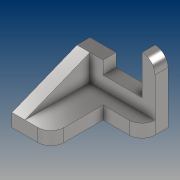
# Autodesk Inventor part: 5
Saved by Autodesk Inventor 2020.2 (Build 242310000, 310)
## iProperties
Created: 2020-09-17
Part Number: 5
Material: 鋼、碳鋼
Document SubType Name: Modeling
Designer: user
Density: 7.85 g/cm^3
Appearance: 半拋光
Mass: 308.946 g
Surface Area: 109.81 cm^2
Volume: 39.3562 cm^3
Author: user
Autodesk Inventor part; units mm, degrees
ref_plane "YZ Plane" through (0, 0, 0) normal (1, 0, 0) x (0, 1, 0)
ref_plane "XZ Plane" through (0, 0, 0) normal (0, 1, 0) x (-1, 0, 0)
ref_plane "XY Plane" through (0, 0, 0) normal (0, 0, 1) x (1, 0, 0)
sketch "草圖1" plane through (0, 0, 0) normal (0, 1, 0) x (-1, 0, 0)
  line L0 (0, 0) -> (0, 60)
  line L1 (-60, 10) -> (-60, 0)
  line L2 (-60, 0) -> (0, 0)
  line L3 (0, 60) -> (-20, 60)
  arc A0 (-20, 60) -> (-30, 50) centre (-20, 50) ccw
  line L4 (-30, 50) -> (-30, 20)
  line L5 (-30, 20) -> (-50, 20)
  arc A1 (-50, 20) -> (-60, 10) centre (-50, 10) ccw
  dimension "d0" = 60
  dimension "d1" = 10
  dimension "d2" = 20
  dimension "d3" = 60
  dimension "d4" = 30
  dimension "d5" = 20
  constraints: 12 end point, 4 point on circle, 4 tangent, 2 centre point, 2 horizontal, 2 perpendicular, 2 vertical
  measures "d0" distance of L1.end L0.start
  measures "d1" distance of L1.start L1.end
  measures "d2" distance of L0.end L3.end
  measures "d3" distance of L0.start L0.end
  measures "d4" distance between parallel lines of L0 L4
  measures "d5" distance between parallel lines of L2 L5
extrude "擠出1" add sketch "草圖1" along normal blind 10
sketch "草圖2" plane through (60, 0, 0) normal (0, 0, -1) x (-1, 0, 0)
  line L0 (0, 0) -> (0, 10) projected
  line L1 (0, 10) -> (60, 10) projected
  line L2 (60, 10) -> (60, 0) projected
  line L3 (60, 0) -> (0, 0) projected
  line L4 (0, 10) -> (0, 40)
  arc A0 (10, 50) -> (0, 40) centre (10, 40) ccw
  line L5 (10, 50) -> (10, 20)
  line L6 (10, 20) -> (40, 20)
  line L7 (40, 20) -> (40, 30)
  line L8 (40, 30) -> (60, 30)
  line L9 (60, 30) -> (60, 10)
  dimension "d8" = 30
  dimension "d9" = 20
  dimension "d10" = 10
  dimension "d11" = 20
  dimension "d12" = 50
  constraints: 12 end point, 3 perpendicular, 2 point on circle, 1 centre point, 1 collinear, 1 parallel, 1 point on line, 1 tangent, 1 vertical
  measures "d8" distance between parallel lines of L8 L3
  measures "d9" distance of L7.end L8.end
  measures "d10" distance between parallel lines of L4 L5
  measures "d11" distance between parallel lines of L3 L6
  measures "d12" distance from line of L3 L5.start
extrude "擠出2" add sketch "草圖2" against normal blind 10 contours L4 A0 L5 L6 L7 L8 L9 L1
sketch "草圖3" plane through (0, 0, 0) normal (-1, 0, 0) x (0, 0, 1)
  line L0 (0, 30) -> (10, 30) projected
  line L1 (10, 30) -> (10, 10) projected
  line L2 (10, 10) -> (60, 10) projected
  line L3 (60, 10) -> (60, 0) projected
  line L4 (60, 0) -> (0, 0) projected
  line L5 (0, 0) -> (0, 30) projected
  line L6 (60, 10) -> (10, 30)
  constraints: 2 end point
extrude "擠出3" add sketch "草圖3" against normal blind 10 contours L6 L2 L1
